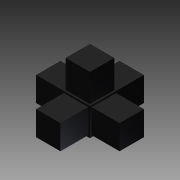
# Autodesk Inventor part: 5-way corner
Saved by Autodesk Inventor 2011 (Build 150239000, 239)
## iProperties
Created: 2013-01-14
Part Number: 5-way corner
Document SubType Name: Modeling
Designer: 351773
Density: 1 g/cm^3
Author: 351773
Autodesk Inventor part; units mm, degrees
ref_plane "YZ Plane" through (0, 0, 0) normal (1, 0, 0) x (0, 1, 0)
ref_plane "XZ Plane" through (0, 0, 0) normal (0, 1, 0) x (-1, 0, 0)
ref_plane "XY Plane" through (0, 0, 0) normal (0, 0, 1) x (1, 0, 0)
sketch "Sketch1" plane through (0, 0, 0) normal (0, 0, 1) x (1, 0, 0)
  line L0 (0, 0) -> (25.4, 0)
  line L1 (25.4, 0) -> (25.4, 25.4)
  line L2 (25.4, 25.4) -> (0, 25.4)
  line L3 (0, 25.4) -> (0, 0)
  line L4 (1.5875, 23.8125) -> (23.8125, 23.8125)
  line L5 (23.8125, 23.8125) -> (23.8125, 1.5875)
  line L6 (23.8125, 1.5875) -> (1.5875, 1.5875)
  line L7 (1.5875, 1.5875) -> (1.5875, 23.8125)
  dimension "d0" = 25.4
  dimension "d1" = 25.4
  dimension "d4" = 1.5875
  constraints: 16 end point, 4 parallel, 2 perpendicular, 1 horizontal, 3 other
  measures "d0" distance of L2.end L1.end
  measures "d1" distance of L1.end L0.end
  measures "d4" distance between parallel lines of L2 L4
extrude "Extrusion1" add sketch "Sketch1" against normal blind 25.4 contours L3 L2 L1 L0 | L4 L5 L6 L7
extrude "Extrusion2" add sketch "Sketch1" along normal blind 25.4 contours L4 L5 L6 L7
sketch "Sketch2" plane through (25.4, 0, 0) normal (1, 0, 0) x (0, 0, -1)
  line L0 (25.4, 0) -> (25.4, 25.4) projected
  line L1 (0, 25.4) -> (25.4, 25.4) projected
  line L2 (0, 0) -> (0, 25.4) projected
  line L3 (0, 0) -> (25.4, 0) projected
  line L4 (23.8125, 23.8125) -> (23.8125, 1.5875)
  line L5 (23.8125, 1.5875) -> (1.5875, 1.5875)
  line L6 (1.5875, 1.5875) -> (1.5875, 23.8125)
  line L7 (1.5875, 23.8125) -> (23.8125, 23.8125)
  dimension "d8" = 1.5875
  constraints: 8 end point, 3 other
  measures "d8" distance between parallel lines of L1 L7
sketch "Sketch3" plane through (0, 25.4, 0) normal (0, 1, 0) x (1, 0, 0)
  line L0 (25.4, 25.4) -> (0, 25.4) projected
  line L1 (0, 0) -> (0, 25.4) projected
  line L2 (25.4, 0) -> (0, 0) projected
  line L3 (25.4, 0) -> (25.4, 25.4) projected
  line L4 (1.5875, 23.8125) -> (23.8125, 23.8125)
  line L5 (23.8125, 23.8125) -> (23.8125, 1.5875)
  line L6 (23.8125, 1.5875) -> (1.5875, 1.5875)
  line L7 (1.5875, 1.5875) -> (1.5875, 23.8125)
  dimension "d9" = 1.5875
  constraints: 8 end point, 3 other
  measures "d9" distance between parallel lines of L0 L4
extrude "Extrusion3" add sketch "Sketch2" along normal blind 25.4 contours L4 L5 L6 L7
extrude "Extrusion4" add sketch "Sketch3" along normal blind 25.4 contours L4 L5 L6 L7
sketch "Sketch4" plane through (0, 0, 0) normal (-1, 0, 0) x (0, 0, 1)
  line L0 (-25.4, 25.4) -> (-25.4, 0) projected
  line L1 (0, 0) -> (-25.4, 0) projected
  line L2 (0, 25.4) -> (0, 0) projected
  line L3 (0, 25.4) -> (-25.4, 25.4) projected
  line L4 (-23.8125, 23.8125) -> (-23.8125, 1.5875)
  line L5 (-23.8125, 1.5875) -> (-1.5875, 1.5875)
  line L6 (-1.5875, 1.5875) -> (-1.5875, 23.8125)
  line L7 (-1.5875, 23.8125) -> (-23.8125, 23.8125)
  dimension "d15" = 1.5875
  constraints: 8 end point, 3 other
  measures "d15" distance between parallel lines of L3 L7
extrude "Extrusion5" add sketch "Sketch4" along normal blind 25.4 contours L7 L6 L5 L4
sketch "Sketch5" plane through (0, 0, -25.4) normal (0, 0, -1) x (-1, 0, 0)
  line L0 (-25.4, 0) -> (-25.4, 25.4) projected
  line L1 (0, 0) -> (-25.4, 0) projected
  line L2 (0, 25.4) -> (0, 0) projected
  line L3 (-25.4, 25.4) -> (0, 25.4) projected
  line L4 (-1.5875, 23.8125) -> (-1.5875, 1.5875)
  line L5 (-1.5875, 1.5875) -> (-23.8125, 1.5875)
  line L6 (-23.8125, 1.5875) -> (-23.8125, 23.8125)
  line L7 (-23.8125, 23.8125) -> (-1.5875, 23.8125)
  dimension "d18" = 1.5875
  constraints: 8 end point, 3 other
  measures "d18" distance between parallel lines of L3 L7
extrude "Extrusion6" add sketch "Sketch5" along normal blind 25.4 contours L4 L5 L6 L7
body "Solid1"
